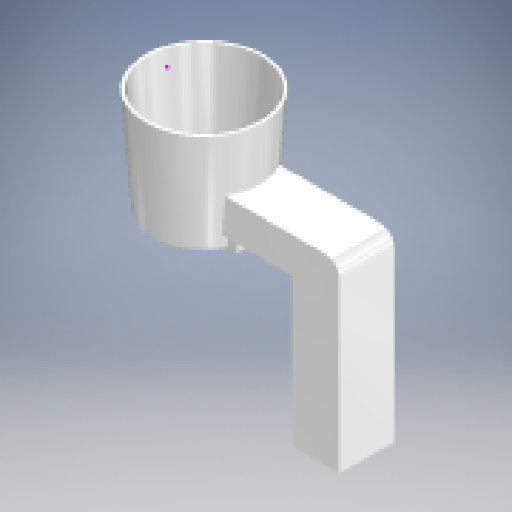
# Autodesk Inventor part: Part3
Saved by Autodesk Inventor 2025.3 (Build 293356000, 356)
## iProperties
Created: 2026-03-06
Part Number: Part3
Material: ABS Plastic
Document SubType Name: Modeling
Designer: Youssef Makhlouf
Density: 1.06 g/cm^3
Appearance: Smooth - White
Author: Youssef Makhlouf
Autodesk Inventor part; units mm, degrees
ref_plane "Work Plane6" through (0, 70, 0) normal (0, 1, 0) x (1, 0, 0)
sketch "Sketch3" plane through (0, 70, 0) normal (0, 1, 0) x (1, 0, 0)
  point P0 (0, 0)
sketch "Sketch5" plane through (0, 0, 0) normal (0, 0, 1) x (1, 0, 0)
  point P0 (0, 0)
ref_plane "Work Plane1" through (120, 0, 0) normal (1, 0, 0) x (0, 1, 0)
sketch "Sketch10" plane through (120, 0, 0) normal (1, 0, 0) x (0, 1, 0)
  line L0 (0, -50) -> (0, 50) projected
  line L1 (0, 15.95) -> (29.7, 15.95)
  line L2 (29.7, 15.95) -> (29.7, -15.95)
  line L3 (29.7, -15.95) -> (0, -15.95)
  line L4 (0, -15.95) -> (0, 15.95)
  line L5 (-14.3752, 0) -> (84.0625, 0) projected
  point P0 (0, 0)
  dimension "d23" = 31.9
  dimension "d24" = 29.7
  constraints: 8 end point, 2 parallel, 1 horizontal, 1 perpendicular, 1 point on line, 1 other
  measures "d23" distance of L1.end L2.end
  measures "d24" distance of L2.end L3.end
extrude "Extrusion6" [suppressed]
ref_plane "Work Plane11" through (0, 0, 0) normal (0, -1, 0) x (1, 0, 0)
sketch "Sketch11" plane through (0, 0, 0) normal (0, -1, 0) x (1, 0, 0)
  circle A0 centre (0, 0) radius 48
  constraints: 1 centre point, 1 coincident
extrude "Extrusion7" [suppressed]
ref_plane "Work Plane10" through (0, 0, 0) normal (0, -1, 0) x (1, 0, 0)
sketch "Sketch12" plane through (0, 0, 0) normal (0, -1, 0) x (1, 0, 0)
  point P0 (0, 0)
extrude "Extrusion8" add sketch "Sketch10" against normal blind 75
ref_plane "Work Plane14" through (0, 0, 0) normal (0, -1, 0) x (1, 0, 0)
sketch "Sketch13" plane through (0, 0, 0) normal (0, -1, 0) x (1, 0, 0)
  circle A0 centre (0, 0) radius 48
  constraints: 1 centre point, 1 coincident
extrude "Extrusion9" cut sketch "Sketch13" against normal blind 75 draft 25
ref_plane "Work Plane13" through (0, 0, 0) normal (0, -1, 0) x (1, 0, 0)
sketch "Sketch14" plane through (0, 0, 0) normal (0, -1, 0) x (1, 0, 0)
  line L0 (74.8, -11.25) -> (63, -11.25)
  line L1 (63, -11.25) -> (63, 11.25)
  line L2 (63, 11.25) -> (74.8, 11.25)
  line L3 (74.8, 11.25) -> (74.8, -11.25)
  line L4 (-123.1698, 0) -> (160.5283, 0) projected
  arc A0 (47.3877, 15.95) -> (47.3877, -15.95) centre (0, 0) ccw projected
  point P0 (63, 0)
  point P1 (74.8, 0)
  dimension "d33" = 11.8
  dimension "d34" = 22.5
  dimension "d35" = 63
  constraints: 8 end point, 2 parallel, 1 horizontal, 1 perpendicular, 1 other
  measures "d33" distance of L1.end L2.end
  measures "d34" distance of L0.end L1.end
  measures "d35" distance from line of A0.centre L1
extrude "Extrusion10" cut sketch "Sketch14" against normal blind 26.7
ref_plane "Work Plane12" through (0, 0, 0) normal (0, -1, 0) x (1, 0, 0)
sketch "Sketch15" plane through (0, 0, 0) normal (0, -1, 0) x (1, 0, 0)
  line L0 (120, 15.95) -> (47.3877, 15.95) projected
  line L1 (120, -15.95) -> (47.3877, -15.95) projected
  line L2 (78.8, 15.95) -> (120, 15.95)
  line L3 (120, 15.95) -> (120, -15.95)
  line L4 (120, -15.95) -> (78.8, -15.95)
  line L5 (78.8, -15.95) -> (78.8, 15.95)
  line L6 (74.8, 11.25) -> (74.8, -11.25) projected
  point P0 (0, 0)
  dimension "d38" = 4
  constraints: 8 end point, 2 parallel, 1 horizontal, 1 perpendicular, 1 point on line
  measures "d38" distance between parallel lines of L6 L5
extrude "Extrusion11" cut sketch "Sketch15" against normal blind 50
ref_plane "Work Plane21" through (78.8, 0, -15.95) normal (0, 0, -1) x (-1, 0, 0)
sketch "Sketch16" plane through (78.8, 0, -15.95) normal (0, 0, -1) x (-1, 0, 0)
  line L0 (15.8, 0) -> (15.8, 26.7) projected
  line L1 (0, 0) -> (31.4123, 0) projected
  line L2 (4, 0) -> (4, 26.7) projected
  line L3 (4, 26.7) -> (15.8, 26.7) projected
  line L4 (4, 0) -> (4, 8.3)
  line L5 (4, 8.3) -> (15.8, 8.3)
  line L6 (15.8, 0) -> (4, 0)
  point P0 (78.8, 0)
  dimension "d41" = 8.3
  constraints: 6 end point, 2 point on line, 1 parallel, 1 perpendicular
  measures "d41" distance of L2.start L4.end
extrude "Extrusion12" cut sketch "Sketch16" against normal blind 50 contours L1 L2 L5 L0
sketch "Sketch17" plane through (74.8, 26.7, 11.25) normal (0, 0, -1) x (-1, 0, 0)
  point P0 (74.8, -26.7)
ref_plane "Work Plane20" through (78.8, 0, 15.95) normal (1, 0, 0) x (0, 0, -1)
sketch "Sketch18" plane through (78.8, 0, 15.95) normal (1, 0, 0) x (0, 0, -1)
  line L0 (27.2, 8.3) -> (27.2, 26.7) projected
  line L1 (4.7, 8.3) -> (4.7, 26.7) projected
  line L2 (4.7, 26.7) -> (27.2, 26.7) projected
  point P0 (15.95, 0)
ref_plane "Work Plane16" through (0, 26.7, 0) normal (0, -1, 0) x (1, 0, 0)
sketch "Sketch19" plane through (0, 26.7, 0) normal (0, -1, 0) x (1, 0, 0)
  line L0 (63, -11.25) -> (74.8, -11.25) projected
  line L1 (63, -15.95) -> (63, 15.95) projected
  line L2 (74.8, -11.25) -> (63, -11.25)
  line L3 (63, -11.25) -> (63, 11.2688)
  line L4 (63, 11.2688) -> (74.8, 11.2688)
  line L5 (74.8, 11.2688) -> (74.8, -11.25)
  point P0 (0, 0)
  constraints: 8 end point, 2 parallel, 1 horizontal, 1 perpendicular, 1 point on line
extrude "Extrusion13" add sketch "Sketch19" along normal blind 2.5
sketch "Sketch20" plane through (74.8, 8.3, 11.25) normal (0, 0, -1) x (-1, 0, 0)
  line L0 (0, -8.3) -> (0, 0) projected
  line L1 (0, 0) -> (11.8, 0) projected
  line L2 (11.8, 0) -> (11.8, -8.3) projected
  line L3 (-4, -8.3) -> (0, -8.3) projected
  line L4 (-4, 21.4) -> (12.975, 21.4) projected
  line L5 (-4, 21.4) -> (-4, -8.3) projected
  line L6 (11.8, -8.3) -> (27.4123, -8.3) projected
  point P0 (74.8, -8.3)
  constraints: 1 other
ref_plane "Work Plane15" through (63, 0, -15.95) normal (0, 0, -1) x (-1, 0, 0)
sketch "Sketch21" plane through (63, 0, -15.95) normal (0, 0, -1) x (-1, 0, 0)
  line L0 (0, 8.3) -> (0, 24.2) projected
  line L1 (-11.8, 8.3) -> (0, 8.3)
  line L2 (0, 8.3) -> (0, 10.8)
  line L3 (0, 10.8) -> (-11.8, 10.8)
  line L4 (-11.8, 10.8) -> (-11.8, 8.3)
  point P0 (63, 0)
  point P1 (0, 8.3)
  dimension "d46" = 2.5
  constraints: 8 end point, 2 parallel, 1 horizontal, 1 perpendicular, 1 point on line
  measures "d46" distance of L2.end L1.end
extrude "Extrusion14" cut sketch "Sketch21" against normal blind 50
sketch "Sketch22" plane through (0, 24.2, 0) normal (0, -1, 0) x (1, 0, 0)
  point P0 (0, 0)
ref_plane "Work Plane22" through (0, 24.2, 0) normal (0, -1, 0) x (1, 0, 0)
sketch "Sketch23" plane through (0, 24.2, 0) normal (0, -1, 0) x (1, 0, 0)
  line L0 (74.8, 11.25) -> (74.8, -11.25) projected
  line L1 (63, -11.25) -> (63, 11.25) projected
  line L2 (74.8, -11.25) -> (63, -11.25)
  line L3 (63, -11.25) -> (63, 11.25)
  line L4 (63, 11.25) -> (74.8, 11.25)
  line L5 (74.8, 11.25) -> (74.8, -11.25)
  point P0 (0, 0)
  constraints: 8 end point, 2 parallel, 1 horizontal, 1 perpendicular
extrude "Extrusion15" cut sketch "Sketch23" against normal blind 2.5
ref_plane "Work Plane5" through (0, 0, 0) normal (0, -1, 0) x (1, 0, 0)
sketch "Sketch24" plane through (0, 0, 0) normal (0, -1, 0) x (1, 0, 0)
  point P0 (0, 0)
ref_plane "Work Plane8" through (0, 0, 0) normal (0, -1, 0) x (1, 0, 0)
sketch "Sketch25" plane through (0, 0, 0) normal (0, -1, 0) x (1, 0, 0)
  circle A0 centre (0, 0) radius 50
  dimension "d51" = 100
  constraints: 1 centre point, 1 coincident
  measures "d51" diameter of A0
extrude "Extrusion16" cut sketch "Sketch25" against normal blind 100 draft 25
ref_plane "Work Plane4" through (0, 0, 0) normal (0, -1, 0) x (1, 0, 0)
sketch "Sketch26" plane through (0, 0, 0) normal (0, -1, 0) x (1, 0, 0)
  point P0 (0, 0)
ref_plane "Work Plane19" through (78.8, 29.7, 15.95) normal (0, 1, 0) x (1, 0, 0)
ref_plane "Work Plane7" through (0, 0, 0) normal (0, -1, 0) x (1, 0, 0)
sketch "Sketch28" plane through (0, 0, 0) normal (0, -1, 0) x (1, 0, 0)
  circle A0 centre (19.8239, 0) radius 35
  line L0 (-39.883, 0) -> (98.5805, 0) projected
  point P0 (0, 0)
  point P1 (51.0715, 15.7666)
  dimension "d55" = 70
  constraints: 1 point on line, 3 other
ref_plane "Work Plane24" through (0, 0, 0) normal (0, -1, 0) x (1, 0, 0)
sketch "Sketch29" plane through (0, 0, 0) normal (0, -1, 0) x (1, 0, 0)
  arc A0 (47.3877, -15.95) -> (49.7159, -5.3226) centre (0, 0) ccw projected
  line L0 (63, -15.95) -> (47.3877, -15.95) projected
  line L1 (63, -15.95) -> (63, 15.95) projected
  line L2 (63, 15.95) -> (47.3877, 15.95) projected
  arc A1 (49.7159, 5.3226) -> (47.3877, 15.95) centre (0, 0) ccw projected
  arc A2 (49.7159, 5.3226) -> (49.7159, -5.3226) centre (15.123, 0) ccw projected
  circle A3 centre (15.123, 0) radius 33
  dimension "d59" = 66
  constraints: 1 centre point, 1 coincident
  measures "d59" diameter of A3
extrude "Extrusion18" cut sketch "Sketch29" against normal blind 70 draft 25 contours A3
ref_plane "Work Plane23" through (63, 0, 15.95) normal (1, 0, 0) x (0, 0, -1)
sketch "Sketch30" plane through (63, 0, 15.95) normal (1, 0, 0) x (0, 0, -1)
  line L0 (0, 29.7) -> (31.9, 29.7) projected
  line L1 (0, 0) -> (31.9, 0)
  line L2 (31.9, 0) -> (31.9, 29.7)
  line L3 (31.9, 29.7) -> (0, 29.7)
  line L4 (0, 29.7) -> (0, 0)
  point P0 (15.95, 0)
  point P1 (0, 29.7)
  constraints: 8 end point, 2 parallel, 1 horizontal, 1 perpendicular
extrude "Extrusion19" add sketch "Sketch30" against normal blind 20
ref_plane "Work Plane26" through (0, 0, 0) normal (0, -1, 0) x (1, 0, 0)
sketch "Sketch31" plane through (0, 0, 0) normal (0, -1, 0) x (1, 0, 0)
  arc A0 (44.0124, 15.95) -> (44.0124, -15.95) centre (15.123, 0) ccw projected
  circle A1 centre (15.123, 0) radius 33
  point P0 (0, 0)
  point P1 (44.0124, -15.95)
  point P2 (44.0124, 15.95)
  constraints: 1 centre point, 1 coincident, 1 concentric
extrude "Extrusion20" cut sketch "Sketch31" against normal blind 70 draft 25
ref_plane "Work Plane18" through (78.8, 0, -15.95) normal (0, 0, -1) x (-1, 0, 0)
sketch "Sketch32" plane through (78.8, 0, -15.95) normal (0, 0, -1) x (-1, 0, 0)
  point P0 (78.8, 0)
ref_plane "Work Plane25" through (0, 0, 0) normal (0, -1, 0) x (1, 0, 0)
sketch "Sketch33" plane through (0, 0, 0) normal (0, -1, 0) x (1, 0, 0)
  line L0 (77.8, 15.95) -> (74.8, 15.95) projected
  line L1 (76.3, 15.95) -> (78.7431, 15.95)
  line L2 (78.7431, 15.95) -> (78.7431, -15.7775)
  line L3 (78.7431, -15.7775) -> (76.3, -15.7775)
  line L4 (76.3, -15.7775) -> (76.3, 15.95)
  line L5 (78.8, -14.95) -> (78.8, 14.95) projected
  line L6 (74.8, -15.95) -> (77.8, -15.95) projected
  point P0 (0, 0)
  constraints: 8 end point, 2 parallel, 1 horizontal, 1 midpoint, 1 perpendicular
ref_plane "Work Plane3" through (0, 0, 0) normal (0, -1, 0) x (1, 0, 0)
sketch "Sketch34" plane through (0, 0, 0) normal (0, -1, 0) x (1, 0, 0)
  arc A0 (46.7694, 14.95) -> (46.7694, -14.95) centre (15.123, 0) ccw projected
  point P0 (0, 0)
ref_plane "Work Plane2" through (0, 0, 0) normal (0, -1, 0) x (1, 0, 0)
sketch "Sketch35" plane through (0, 0, 0) normal (0, -1, 0) x (1, 0, 0)
  circle A0 centre (15.123, 0) radius 33.6634 projected
  point P0 (0, 0)
ref_plane "Work Plane17" through (78.8, 1, 14.95) normal (1, 0, 0) x (0, 0, -1)
sketch "Sketch36" plane through (78.8, 1, 14.95) normal (1, 0, 0) x (0, 0, -1)
  point P0 (14.95, -1)
ref_plane "Work Plane27" through (15.123, 70, 0) normal (0, 1, 0) x (1, 0, 0)
sketch "Sketch38" plane through (63, 0, -15.95) normal (0, -1, 0) x (1, 0, 0)
  point P0 (-63, 15.95)
sketch "Sketch39" plane through (63, 0, -15.95) normal (0, -1, 0) x (1, 0, 0)
  line L0 (18.7198, 15.95) -> (-64.9525, 15.95)
  line L1 (0, 0) -> (-18.9876, 0) projected
  circle A0 centre (-37.9729, 15.95) radius 35
  point P0 (-63, 15.95)
  dimension "d70" = 15.95
  dimension "d72" = 70
  constraints: 2 end point, 1 centre point, 1 horizontal
  measures "d70" distance between parallel lines of L1 L0
  measures "d72" diameter of A0
sketch "Sketch40" plane through (78.8, 29.7, 15.95) normal (0, 1, 0) x (1, 0, 0)
  point P0 (-78.8, 15.95)
ref_plane "Work Plane28" through (63, 70, -15.95) normal (0, -1, 0) x (1, 0, 0)
sketch "Sketch41" plane through (63, 70, -15.95) normal (0, -1, 0) x (1, 0, 0)
  circle A0 centre (-37.9729, 15.95) radius 35 projected
  circle A1 centre (-37.9729, 15.95) radius 40
  point P0 (-63, 15.95)
  dimension "d74" = 80
  constraints: 1 centre point, 1 coincident
  measures "d74" diameter of A1
sketch "Sketch42" plane through (63, 70, -15.95) normal (0, -1, 0) x (1, 0, 0)
  circle A0 centre (-37.9729, 15.95) radius 35 projected
  circle A1 centre (-37.9729, 15.95) radius 38
  point P0 (-63, 15.95)
  dimension "d75" = 76
  constraints: 1 centre point, 1 coincident
  measures "d75" diameter of A1
sketch "Sketch43" plane through (63, 0, -15.95) normal (0, -1, 0) x (1, 0, 0)
  circle A0 centre (-37.9729, 15.95) radius 35 projected
  circle A1 centre (-37.9729, 15.95) radius 33
  point P0 (-63, 15.95)
  dimension "d76" = 66
  constraints: 1 centre point, 1 coincident
  measures "d76" diameter of A1
loft "Loft1" add profiles "Sketch39", "Sketch41" contours all / A0 | A1
loft "Loft2" cut profiles "Sketch43", "Sketch42" contours A1 / A0 | A1
sketch "Sketch44" plane through (78.8, 29.7, 15.95) normal (0, 1, 0) x (1, 0, 0)
  point P0 (-78.8, 15.95)
sketch "Sketch45" plane through (78.8, 29.7, 15.95) normal (0, 1, 0) x (1, 0, 0)
  arc A0 (-17.4865, 8.1206) -> (-17.4865, 23.7794) centre (-53.7729, 15.95) ccw projected
  arc A1 (-19.6264, 0) -> (-17.4865, 8.1206) centre (-63.677, 15.95) ccw projected
  line L0 (0, 0) -> (-19.6264, 0) projected
  line L1 (0, 0) -> (0, 31.9) projected
  line L2 (0, 31.9) -> (-19.6264, 31.9) projected
  arc A2 (-17.4865, 23.7794) -> (-19.6264, 31.9) centre (-63.677, 15.95) ccw projected
  line L3 (-15.8, 26.3297) -> (-15.8, 5.5703) projected
  arc A3 (-15.8, 5.5703) -> (-15.8, 26.3297) centre (-78.8, 15.95) ccw projected
extrude "Extrusion21" add sketch "Sketch45" against normal blind 1 contours A3 L3
sketch "Sketch47" plane through (74.8, 0, -15.95) normal (0, -1, 0) x (1, 0, 0)
  point P0 (-74.8, 15.95)
sketch "Sketch49" plane through (63, 10.8, -11.25) normal (0, -1, 0) x (1, 0, 0)
  line L0 (5.9, 1.1557) -> (5.9, -5.6707)
  line L1 (8.2413, -2.4) -> (3.9567, -2.4)
  line L2 (11.8, -4.7) -> (0, -4.7) projected
  circle A0 centre (5.9, -2.4) radius 1
  line L3 (19.0031, 11.25) -> (2.8858, 11.25)
  point P0 (-63, 11.25)
  dimension "d95" = 2.3
  dimension "d96" = 2
  constraints: 6 end point, 2 point on line, 1 centre point, 1 horizontal, 1 perpendicular, 1 vertical
  measures "d95" distance between parallel lines of L2 L1
  measures "d96" diameter of A0
sketch "Sketch50" plane through (63, 10.8, 11.25) normal (0, -1, 0) x (1, 0, 0)
  line L0 (5.9, 6.3005) -> (5.9, -1.1655)
  line L1 (9.1451, 2.4) -> (2.8622, 2.4)
  line L2 (0, 4.7) -> (11.8, 4.7) projected
  circle A0 centre (5.9, 2.4) radius 1
  point P0 (-63, -11.25)
  dimension "d97" = 2.3
  dimension "d98" = 2
  constraints: 4 end point, 2 point on line, 1 centre point, 1 horizontal, 1 vertical
  measures "d97" distance between parallel lines of L2 L1
  measures "d98" diameter of A0
extrude "Extrusion23" cut sketch "Sketch50" against normal blind 8
extrude "Extrusion24" cut sketch "Sketch49" against normal blind 8
sketch "Sketch51" plane through (78.8, 0, 15.95) normal (1, 0, 0) x (0, 0, -1)
  line L0 (4.7, 10.8) -> (4.7, 26.7) projected
  line L1 (27.2, 10.8) -> (27.2, 26.7) projected
  line L2 (4.7, 26.7) -> (27.2, 26.7) projected
  line L3 (31.9, 10.8) -> (27.2, 10.8) projected
  line L4 (4.7, 26.7) -> (27.2, 26.7)
  line L5 (27.2, 26.7) -> (27.2, 10.8)
  line L6 (27.2, 10.8) -> (4.7, 10.8)
  line L7 (4.7, 10.8) -> (4.7, 26.7)
  point P0 (15.95, 0)
  constraints: 8 end point, 2 parallel, 1 horizontal, 1 perpendicular
extrude "Extrusion25" cut sketch "Sketch51" against normal blind 5
sketch "Sketch52" plane through (78.8, 0, 15.95) normal (1, 0, 0) x (0, 0, -1)
  line L0 (27.2, 10.8) -> (4.7, 10.8) projected
  line L1 (0, 0) -> (31.9, 0) projected
  line L2 (4.7, 10.8) -> (27.2, 10.8)
  line L3 (27.2, 10.8) -> (27.2, 0)
  line L4 (27.2, 0) -> (4.7, 0)
  line L5 (4.7, 0) -> (4.7, 10.8)
  point P0 (15.95, 0)
  constraints: 8 end point, 2 parallel, 1 horizontal, 1 perpendicular, 1 point on line
extrude "Extrusion26" cut sketch "Sketch52" against normal blind 5
sketch "Sketch53" plane through (78.8, 0, -15.95) normal (1, 0, 0) x (0, 0, -1)
  line L0 (0, 10.8) -> (-4.7, 10.8) projected
  line L1 (-27.2, 10.8) -> (-31.9, 10.8) projected
  line L2 (-31.9, 10.8) -> (-31.9, 0) projected
  line L3 (-31.9, 0) -> (0, 0)
  line L4 (0, 0) -> (0, 10.8)
  line L5 (0, 10.8) -> (-31.9, 10.8)
  line L6 (-31.9, 10.8) -> (-31.9, 0)
  point P0 (-15.95, 0)
  constraints: 8 end point, 2 parallel, 1 horizontal, 1 perpendicular
extrude "Extrusion27" cut sketch "Sketch53" against normal blind 5
sketch "Sketch54" plane through (63, 10.8, -11.25) normal (0, -1, 0) x (1, 0, 0)
  line L0 (15.8, 0) -> (0, 0) projected
  line L1 (15.8, 0) -> (0, 0)
  line L2 (0, 0) -> (0, -0.5)
  line L3 (0, -0.5) -> (15.8, -0.5)
  line L4 (15.8, -0.5) -> (15.8, 0)
  line L5 (17.1839, 11.25) -> (-1.6865, 11.25)
  point P0 (-63, 11.25)
  dimension "d109" = 0.5
  constraints: 10 end point, 2 horizontal, 2 parallel, 1 perpendicular
  measures "d109" distance of L2.end L1.end
extrude "Extrusion28" cut sketch "Sketch54" against normal blind 15.9
sketch "Sketch55" plane through (63, 10.8, 15.95) normal (0, -1, 0) x (1, 0, 0)
  line L0 (15.8, -4.7) -> (0, -4.7) projected
  line L1 (0, -31.9) -> (0, 0) projected
  line L2 (15.8, -4.7) -> (0, -4.7)
  line L3 (0, -4.7) -> (0, -4.2)
  line L4 (0, -4.2) -> (15.8, -4.2)
  line L5 (15.8, -4.2) -> (15.8, -4.7)
  point P0 (-63, -15.95)
  dimension "d112" = 0.5
  constraints: 8 end point, 2 parallel, 1 horizontal, 1 perpendicular, 1 point on line
  measures "d112" distance of L2.end L3.end
extrude "Extrusion29" cut sketch "Sketch55" against normal blind 15.9
sketch "Sketch56" plane through (78.8, 29.7, 15.95) normal (1, 0, 0) x (0, 0, -1)
  line L0 (4.2, -18.9) -> (4.2, -3) projected
  line L1 (4.2, -3) -> (27.7, -3) projected
  line L2 (27.7, -3) -> (27.7, -18.9) projected
  line L3 (27.7, -18.9) -> (31.9, -18.9) projected
  line L4 (31.9, 0) -> (31.9, -18.9) projected
  line L5 (0, 0) -> (31.9, 0) projected
  line L6 (0, -18.9) -> (0, 0) projected
  line L7 (0, -18.9) -> (4.2, -18.9) projected
  point P0 (15.95, -29.7)
sketch "Sketch57" plane through (78.8, 10.8, -15.95) normal (0, 0, -1) x (-1, 0, 0)
  line L0 (0, 0) -> (0, 18.9) projected
  line L1 (0, 0) -> (15.8, 0) projected
  line L2 (0, 18.9) -> (3.8, 18.9)
  line L3 (3.8, 18.9) -> (3.8, 0)
  line L4 (3.8, 0) -> (0, 0)
  line L5 (0, 0) -> (0, 18.9)
  point P0 (78.8, -10.8)
  dimension "d115" = 3.8
  constraints: 8 end point, 2 parallel, 1 horizontal, 1 perpendicular, 1 point on line
  measures "d115" distance of L3.end L4.end
extrude "Extrusion30" cut sketch "Sketch57" against normal blind 50
sketch "Sketch58" plane through (63, 10.8, -15.95) normal (0, -1, 0) x (1, 0, 0)
  point P0 (-63, 15.95)
sketch "Sketch59" plane through (63, 10.8, -15.95) normal (0, -1, 0) x (1, 0, 0)
  line L0 (12, 4.2) -> (12, 27.7) projected
  line L1 (0, 0) -> (0, 31.9) projected
  line L2 (12, 4.2) -> (0, 4.2)
  line L3 (0, 4.2) -> (0, 3.7)
  line L4 (0, 3.7) -> (12, 3.7)
  line L5 (12, 3.7) -> (12, 4.2)
  line L6 (12, 31.9) -> (12, 0) projected
  line L7 (0, 27.7) -> (12, 27.7)
  line L8 (12, 27.7) -> (12, 28.2)
  line L9 (12, 28.2) -> (0, 28.2)
  line L10 (0, 28.2) -> (0, 27.7)
  point P0 (-63, 15.95)
  point P1 (0, 4.2)
  dimension "d118" = 0.5
  dimension "d119" = 0.5
  constraints: 16 end point, 4 parallel, 3 point on line, 2 horizontal, 2 perpendicular
  measures "d118" distance of L3.end L2.end
  measures "d119" distance of L8.end L7.end
extrude "Extrusion31" cut sketch "Sketch59" against normal blind 15.9 contours L5 L4 L1 L2 | L7 L1 L9 L6
sketch "Sketch60" plane through (75, 10.8, -15.95) normal (1, 0, 0) x (0, 0, -1)
  line L0 (-31.9, 18.9) -> (0, 18.9) projected
  line L1 (-31.9, 0) -> (0, 0)
  line L2 (0, 0) -> (0, 18.9)
  line L3 (0, 18.9) -> (-31.9, 18.9)
  line L4 (-31.9, 18.9) -> (-31.9, 0)
  line L5 (-31.9, 0) -> (0, 18.9) construction
  line L6 (0, 0) -> (-31.9, 18.9) construction
  line L7 (-34.4, -2.5) -> (2.5, -2.5)
  line L8 (2.5, -2.5) -> (2.5, 21.4)
  line L9 (2.5, 21.4) -> (-34.4, 21.4)
  line L10 (-34.4, 21.4) -> (-34.4, -2.5)
  point P0 (-15.95, -10.8)
  point P1 (-15.95, 9.45)
  dimension "d122" = 2.5
  constraints: 20 end point, 4 parallel, 2 midpoint, 2 perpendicular, 1 horizontal, 3 other
  measures "d122" distance between parallel lines of L4 L10
extrude "Extrusion32" add sketch "Sketch60" along normal blind 60 and the other way blind 20
sketch "Sketch61" plane through (135, 10.8, -15.95) normal (1, 0, 0) x (0, 0, -1)
  line L0 (0, -2.5) -> (0, -10.8) projected
  line L1 (-31.5106, 0) -> (-0.3894, 0) projected
  line L2 (0, -2.5) -> (-31.5106, -2.5)
  line L3 (-31.5106, -2.5) -> (-31.5106, 0)
  line L4 (-31.5106, 0) -> (0, 0)
  line L5 (0, 0) -> (0, -2.5)
  point P0 (-15.95, -10.8)
  constraints: 8 end point, 2 parallel, 1 horizontal, 1 perpendicular
extrude "Extrusion33" cut sketch "Sketch61" against normal blind 60
extrude "Extrusion34" add sketch "Sketch61" against normal blind 60
sketch "Sketch62" plane through (55.4647, 8.3, 18.45) normal (0, -1, 0) x (1, 0, 0)
  line L0 (51.0353, -5.95) -> (76.0353, -5.95)
  line L1 (76.0353, -5.95) -> (76.0353, -30.95)
  line L2 (76.0353, -30.95) -> (51.0353, -30.95)
  line L3 (51.0353, -30.95) -> (51.0353, -5.95)
  line L4 (51.0353, -5.95) -> (76.0353, -30.95) construction
  line L5 (76.0353, -5.95) -> (51.0353, -30.95) construction
  line L6 (79.5353, 0) -> (79.5353, -36.9) projected
  line L7 (1.9798, -36.9) -> (79.5353, -36.9) projected
  line L8 (47.5353, 0) -> (79.5353, 0)
  line L9 (79.5353, 0) -> (79.5353, -36.9)
  line L10 (79.5353, -36.9) -> (47.5353, -36.9)
  line L11 (47.5353, -36.9) -> (47.5353, 0)
  line L12 (47.5353, 0) -> (79.5353, -36.9) construction
  line L13 (79.5353, 0) -> (47.5353, -36.9) construction
  point P0 (-55.4647, -18.45)
  point P1 (63.5353, -18.45)
  point P2 (79.5353, -18.45)
  dimension "d131" = 25
  dimension "d132" = 25
  dimension "d133" = 3.5
  constraints: 24 end point, 5 midpoint, 4 parallel, 2 horizontal, 2 perpendicular, 1 horizontal alignment
  measures "d131" distance of L1.end L2.end
  measures "d132" distance of L0.end L1.end
  measures "d133" distance between parallel lines of L1 L6
extrude "Extrusion35" cut sketch "Sketch62" against normal blind 10 contours L0 L1 L2 L3
extrude "Extrusion36" add sketch "Sketch62" along normal blind 108
sketch "Sketch63" plane through (75, 10.8, 15.95) normal (0, 1, 0) x (1, 0, 0)
  line L0 (60, 31.9) -> (56.5, 31.9)
  line L1 (56.5, 31.9) -> (56.5, 0)
  line L2 (56.5, 0) -> (60, 0)
  line L3 (60, 0) -> (60, 31.9)
  point P0 (-75, 15.95)
  dimension "d138" = 3.5
  constraints: 8 end point, 2 parallel, 1 horizontal, 1 perpendicular
  measures "d138" distance of L2.end L1.end
extrude "Extrusion37" add sketch "Sketch63" along normal up to surface (21.4 mm away)
fillet "Fillet4" radius 10 1 edges at (135, 32.2, 0)
body "Solid1"
